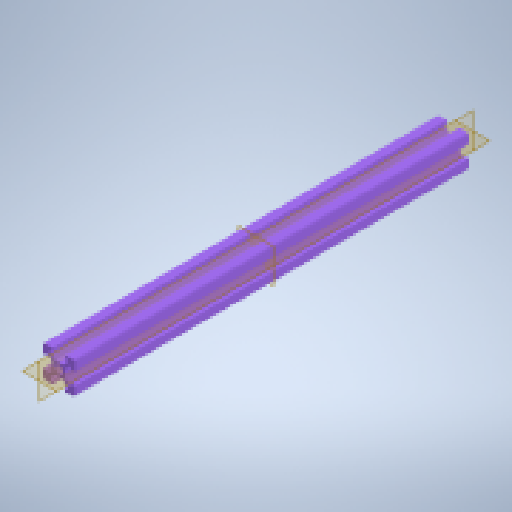
# Autodesk Inventor part: Peça2
Saved by Autodesk Inventor 2025.2 (Build 292293000, 293)
## iProperties
Created: 2025-03-25
Part Number: Peça2
Material: Aço
Document SubType Name: Modeling
Designer: Formação
Density: 7.85 g/cm^3
Appearance: Violeta
Author: Formação
Autodesk Inventor part; units mm, degrees
sketch "Esboço1" plane through (0, 0, 0) normal (0, 0, 1) x (1, 0, 0)
  line L0 (-10, 10) -> (10, 10) construction
  circle A0 centre (0, 0) radius 2.5 construction
  line L1 (-4, 4) -> (4, 4) construction
  line L2 (-4, 4) -> (-4, -4) construction
  line L3 (-10, 10) -> (0, 0) construction
  line L4 (-2.5858, 4) -> (-6.5858, 8) construction
  line L5 (-6.5858, 8) -> (0, 8) construction
  arc A1 (-5.3787, 8) -> (-5.7322, 7.1464) centre (-5.3787, 7.5) ccw
  arc A2 (-2.7322, 4.1464) -> (-2.3787, 4) centre (-2.3787, 4.5) ccw
  line L6 (0, 4) -> (-4, 4) construction
  line L7 (-2.3787, 4) -> (0, 4)
  line L8 (-4, 10) -> (-4, 8) construction
  line L9 (-5.3787, 8) -> (-4, 8)
  line L10 (-5.7322, 7.1464) -> (-2.7322, 4.1464)
  line L11 (-4, 10) -> (-4, 9) construction
  line L12 (-4, 9) -> (-4, 9) construction
  line L13 (-4, 10) -> (-4, 9)
  line L14 (-4, 9) -> (-4, 9)
  line L15 (-4, 9) -> (-4, 8)
  line L16 (0, 4) -> (0, 2.5)
  arc A3 (-9, 10) -> (-9.7071, 9.7071) centre (-9, 9) ccw
  line L17 (-9, 10) -> (-4, 10)
  line L18 (-9.7071, 9.7071) -> (-1.7678, 1.7678)
  arc A4 (0, 2.5) -> (-1.7678, 1.7678) centre (0, 0) ccw
  point P0 (0, 10)
  point P1 (-4, 0)
  point P2 (-5, 5)
  point P3 (-5.8406, 7.6913)
  point P4 (-9.3827, 9.9239)
  point P5 (-6.5, 10)
  dimension "d1" = 10
  dimension "d2" = 5
  dimension "d5" = 20
  dimension "d10" = 1
  dimension "d11" = 2
  dimension "d17" = 6
  dimension "d18" = 0.5
  dimension "d24" = 1
  dimension "d25" = 0.5
  constraints: 38 end point, 12 point on circle, 9 point on line, 7 midpoint, 6 horizontal, 5 centre point, 5 collinear, 5 tangent, 5 vertical alignment, 4 perpendicular, 3 horizontal alignment, 2 coincident, 2 vertical, 1 line through centre, 1 parallel
  measures "d1" horizontal distance of point (0, 0) L0.start
  measures "d2" diameter of A0
  measures "d5" distance of L0.end L0.start
  measures "d10" distance from line of point (-5, 5) L4
  measures "d11" distance from line of L4.end L0
  measures "d17" distance between parallel lines of L0 L1
  measures "d18" radius of A2
  measures "d24" radius of A3
  measures "d25" radius of A1
extrude "Extrusão1" add sketch "Esboço1" along normal mid plane 250
mirror "Espelhar1" about plane through (-9.7071, 9.7071, 0) normal (-0.7071, -0.7071, 0)
mirror "Espelhar2" about plane through (0, 0, 0) normal (1, 0, 0)
mirror "Espelhar3" about plane through (0, 0, 0) normal (0, 1, 0)
